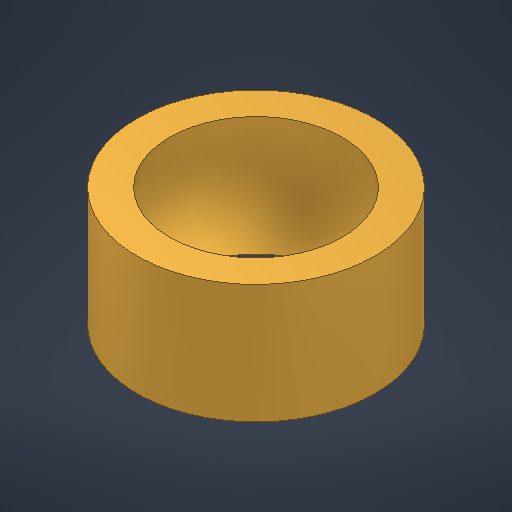
# Autodesk Inventor part: Cylinder
Saved by Autodesk Inventor 2025 (Build 290162000, 162)
## iProperties
Created: 2024-10-17
Part Number: Cylinder
Material: Латунь, мягкая, желтая
Document SubType Name: Modeling
Designer: khrip
Density: 8.47 g/cm^3
Appearance: Латунь — сатинированная
Author: khrip
Autodesk Inventor part; units mm, degrees
ref_plane "YZ Plane" through (0, 0, 0) normal (1, 0, 0) x (0, 1, 0)
ref_plane "XZ Plane" through (0, 0, 0) normal (0, 1, 0) x (-1, 0, 0)
ref_plane "XY Plane" through (0, 0, 0) normal (0, 0, 1) x (1, 0, 0)
sketch "Эскиз1" plane through (0, 0, 0) normal (0, 1, 0) x (-1, 0, 0)
  circle A0 centre (0, 0) radius 4.5
  dimension "d0" = 9
  constraints: 1 centre point, 1 coincident
  measures "d0" diameter of A0
extrude "Выдавливание1" add sketch "Эскиз1" along normal mid plane 4.5
sketch "Эскиз2" plane through (0, 0, 0) normal (0, 1, 0) x (-1, 0, 0)
  circle A0 centre (0, 0) radius 3.969
  line L0 (3.969, 0) -> (-3.969, 0)
  dimension "d3" = 7.938
  dimension "d4" = 7.938
  constraints: 2 end point, 2 point on circle, 1 centre point, 1 coincident, 1 horizontal
  measures "d3" diameter of A0
  measures "d4" distance of L0.start L0.end
revolve "Вращение1" cut sketch "Эскиз2" angle 360 about axis through (-3.969, 0, 0) along (1, 0, 0) picked at (1.323, -1.2297) contours A0 L0
